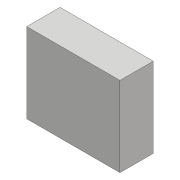
# Autodesk Inventor part: ldr_case
Saved by Autodesk Inventor 2018 (Build 220112000, 112)
## iProperties
Created: 2017-08-12
Part Number: ldr_case
Material: Generic
Document SubType Name: Modeling
Designer: isaacporras
Density: 1 g/cm^3
Appearance: Default
Author: isaacporras
Autodesk Inventor part; units mm, degrees
ref_plane "YZ Plane" through (0, 0, 0) normal (1, 0, 0) x (0, 1, 0)
ref_plane "XZ Plane" through (0, 0, 0) normal (0, 1, 0) x (-1, 0, 0)
ref_plane "XY Plane" through (0, 0, 0) normal (0, 0, 1) x (1, 0, 0)
sketch "Sketch1" plane through (0, 0, 0) normal (0, 1, 0) x (-1, 0, 0)
  line L0 (7, 6) -> (-7, 6)
  line L1 (-7, 6) -> (-7, -6)
  line L2 (-7, -6) -> (7, -6)
  line L3 (7, -6) -> (7, 6)
  line L4 (7, 6) -> (-7, -6) construction
  line L5 (-7, 6) -> (7, -6) construction
  line L6 (4.3106, 4.4) -> (1.6094, 4.4) construction
  line L7 (1.6094, 4.4) -> (1.6094, 0.23) construction
  line L8 (1.6094, 0.23) -> (4.3106, 0.23) construction
  line L9 (4.3106, 0.23) -> (4.3106, 4.4) construction
  line L10 (4.3106, 4.4) -> (1.6094, 0.23) construction
  line L11 (1.6094, 4.4) -> (4.3106, 0.23) construction
  arc A0 (4.3106, 0.23) -> (4.3106, 4.4) centre (2.86, 2.315) ccw construction
  arc A1 (1.6094, 4.4) -> (1.6094, 0.23) centre (3.06, 2.315) ccw construction
  point P0 (0, 0)
  point P1 (2.96, 2.315)
  dimension "d0" = 12
  dimension "d1" = 14
  dimension "d2" = 4.17
  dimension "d3" = 2.54
  dimension "d4" = 4.88
  dimension "d6" = 1.6
  dimension "d7" = 1.6
  constraints: 24 end point, 4 midpoint, 4 parallel, 4 point on circle, 2 centre point, 2 horizontal, 2 perpendicular, 1 equal radius
  measures "d0" distance of L2.end L0.start
  measures "d1" distance of L1.end L2.end
  measures "d2" distance of L8.end L6.start
  measures "d3" radius of A0
  measures "d6" distance between parallel lines of L0 L6
  measures "d7" distance edge to line of A0 L3
extrude "Extrusion1" add sketch "Sketch1" against normal blind 5
sketch "Sketch2" plane through (0, 0, 0) normal (0, 1, 0) x (1, 0, 0)
  line L0 (-4.3106, -4.4) -> (-1.6094, -4.4) construction
  arc A0 (-4.3106, -0.23) -> (-4.3106, -4.4) centre (-2.86, -2.315) ccw construction
  arc A1 (-1.6094, -4.4) -> (-1.6094, -0.23) centre (-3.06, -2.315) ccw construction
  arc A2 (-4.8304, 0) -> (-4.4598, -4.9) centre (-2.86, -2.315) ccw
  line L1 (-4.4598, -4.9) -> (-1.4602, -4.9)
  arc A3 (-1.4602, -4.9) -> (-0.02, -2.315) centre (-3.06, -2.315) ccw
  line L2 (-7, 6) -> (-7, -6) projected
  line L3 (-7, -6) -> (7, -6) projected
  line L4 (-4.8304, 0) -> (-6.4599, 0)
  line L5 (-6.4599, 0) -> (-6.4599, -5.558) construction
  line L6 (-6.4599, -5.558) -> (0, -5.558) construction
  line L7 (0, -5.558) -> (0, -2.315) construction
  line L8 (0, -2.315) -> (-0.02, -2.315)
  line L9 (0, 8.4) -> (0, -8.4) projected
  line L10 (0, -2.315) -> (0, 0)
  line L11 (-4.8304, 0) -> (0, 0)
  dimension "d10" = 0.5
  constraints: 16 end point, 4 perpendicular, 4 point on circle, 2 centre point, 2 collinear, 2 horizontal
  measures "d10" radial gap between concentric circles of A0 A2
extrude "Extrusion2" cut sketch "Sketch2" against normal blind 2
mirror "Mirror1" about plane through (0, 0, 0) normal (0, 0, 1) of "Extrusion2"
mirror "Mirror2" about plane through (0, 0, 0) normal (1, 0, 0) of "Extrusion2", "Mirror1"
fillet "Fillet1" radius 0.25 6 edges at (-4.8304, -1, 0) (0.02, -1, 2.315) (0.02, -1, -2.315) (-0.02, -1, 2.315) (-0.02, -1, -2.315) (4.8304, -1, 0)
body "Solid1"
